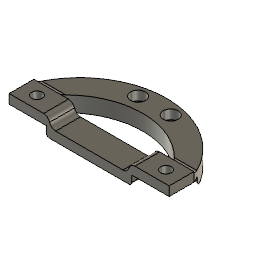
mount v6 (Autodesk Fusion 360 design; units mm, degrees)
Autodesk Fusion 360 part; units mm, degrees
note: some values were not read from the file. Chosen so that the rebuilt part matches the saved one: which bodies a step acts on.
sketch "Sketch1" plane through (0, 0, 0) normal (0, 0, 1) x (1, 0, 0)
  line L0 (0, 0) -> (51.5, 0)
  line L1 (51.5, 0) -> (51.5, 8)
  line L2 (51.5, 8) -> (0, 8)
  line L3 (0, 8) -> (0, 0)
  circle A0 centre (5, 4) radius 1.7
  circle A1 centre (46.5, 4) radius 1.7
  circle A2 centre (20.5, 21) radius 2.4
  circle A3 centre (31, 21) radius 2.4
  arc A4 (51.5, 8) -> (0, 8) centre (25.75, -2.9486) ccw
  arc A5 (45, 8) -> (7, 8) centre (26, -7.6356) ccw
  circle A6 centre (20.5, 21) radius 1.8
  circle A7 centre (31, 21) radius 1.8
  dimension "d1" = 51.5
  dimension "d2" = 8
  dimension "d3" = 3.4
  dimension "d4" = 5
  dimension "d5" = 4
  dimension "d6" = 3.4
  dimension "d7" = 5
  dimension "d8" = 4
  dimension "d9" = 4.8
  dimension "d10" = 17
  dimension "d11" = 4.8
  dimension "d12" = 17
  dimension "d13" = 10.5
  dimension "d14" = 15.5
  dimension "d15" = 3.6
  dimension "d16" = 3.6
  constraint horizontal L0
  constraint vertical L1
  constraint horizontal L2
  constraint vertical L3
  constraint coincident L0.start L3.end
  constraint coincident L2 A5.start
  constraint coincident L2 A5.end
  constraint concentric A2 A6
  constraint concentric A3 A7
  measures "d1" distance of L0.start L0.end
  measures "d2" distance of L0.start L2.end
  measures "d3" diameter of A0
  measures "d4" distance of L3 A0.centre
  measures "d5" distance of L0 A0.centre
  measures "d6" diameter of A1
  measures "d7" distance of L1 A1.centre
  measures "d8" distance of L0 A1.centre
  measures "d9" diameter of A2
  measures "d10" vertical distance of A0.centre A2.centre
  measures "d11" diameter of A3
  measures "d12" vertical distance of A1.centre A3.centre
  measures "d13" distance of A2.centre A3.centre
  measures "d14" horizontal distance of A0.centre A2.centre
  measures "d15" diameter of A6
  measures "d16" diameter of A7
extrude "Extrude1" add sketch "Sketch1" along normal blind 2 contours A2 makes body 1
extrude "Extrude2" [suppressed]
extrude "Extrude3" add sketch "Sketch1" along normal blind 2 contours A3 bodies 1 makes body 2
extrude "Extrude4" add sketch "Sketch1" along normal blind 3 contours L0 L1 L2 L3 bodies 1 makes body 3
fillet "Fillet1" [suppressed]
fillet "Fillet2" [suppressed]
sketch "Sketch3" plane through (0, 0, 3) normal (0, 0, 1) x (-1, 0, 0)
  line L0 (-51.5, 0) -> (-51.5, -8)
  line L1 (-51.5, -8) -> (0, -8)
  line L2 (0, -8) -> (0, 0)
  line L3 (0, 0) -> (-51.5, 0)
  circle A0 centre (-5, -4) radius 1.7
  circle A1 centre (-46.5, -4) radius 1.7
  line L4 (-13, -8) -> (-38.5, -8)
  line L5 (-38.5, -8) -> (-38.5, 0)
  line L6 (-38.5, 0) -> (-13, 0)
  line L7 (-13, 0) -> (-13, -8)
  point P0 (-5, -4)
  point P1 (-46.5, -4)
  dimension "d29" = 8
  dimension "d30" = 8
  constraint horizontal L4
  constraint vertical L5
  constraint horizontal L6
  constraint vertical L7
  constraint coincident L3 L5.end
  measures "d29" distance of L7 P0
  measures "d30" distance of L5 P1
extrude "Extrude5" cut sketch "Sketch3" against normal blind 3 contours L1 L3 L4 L5 L6 L7 bodies 3 makes body 4 at (10.9, 4, 0)
sketch "Sketch5" plane through (0, 0, 0) normal (0, 0, 1) x (1, 0, 0)
  line L0 (12, 0) -> (39.5, 0)
  line L1 (39.5, 0) -> (39.5, 8)
  line L2 (39.5, 8) -> (12, 8)
  line L3 (12, 8) -> (12, 0)
  point P0 (5, 4)
  point P1 (46.5, 4)
  dimension "d35" = 7
  dimension "d36" = 7
  constraint horizontal L0
  constraint vertical L1
  constraint horizontal L2
  constraint vertical L3
  measures "d35" distance of L3 P0
  measures "d36" distance of L1 P1
extrude "Extrude6" add sketch "Sketch5" against normal blind 3 bodies 1 2 3 4
fillet "Fillet3" radius 2 4 edges at (13, 4, 0) (13, 4, 3) (38.5, 4, 3) (38.5, 4, 0) on bodies 3
fillet "Fillet4" radius 1 2 edges at (39.5, 4, -3) (12, 4, -3) on bodies 3
extrude "Extrude7" add sketch "Sketch1" against normal blind 3 separate body contours L2 A4 A5 makes body 5
extrude "Extrude8" add sketch "Sketch1" against normal blind 3 contours A2 | A3 bodies 5
extrude "Extrude9" cut sketch "Sketch1" against normal blind 1 contours A2 | A3 bodies 5
extrude "Extrude10" add sketch "Sketch1" along normal blind 2 contours L2 A4 A5 bodies 3 5
extrude "Extrude11" cut 2 faces at (49.3333, 8, -1) (4.6667, 8, -1) along direction (0, 1, 0) blind 2 on bodies 3 bodies 3
fillet "Fillet5" [suppressed]
fillet "Fillet6" radius 2 2 edges at (48.25, 8, 2) (3.5, 8, 2) on bodies 3
extrude "Extrude12" cut 1 faces at (7, 8.6667, -1) along direction (1, 0, 0) blind 2 on bodies 3 bodies 3
extrude "Extrude13" cut 1 faces at (45, 8.6667, -1) along direction (-1, 0, 0) blind 2 on bodies 3 bodies 3
fillet "Fillet7" radius 2 2 edges at (4.8928, 10, -3) (46.8572, 10, -3) on bodies 3
hidden bodies 1 2
